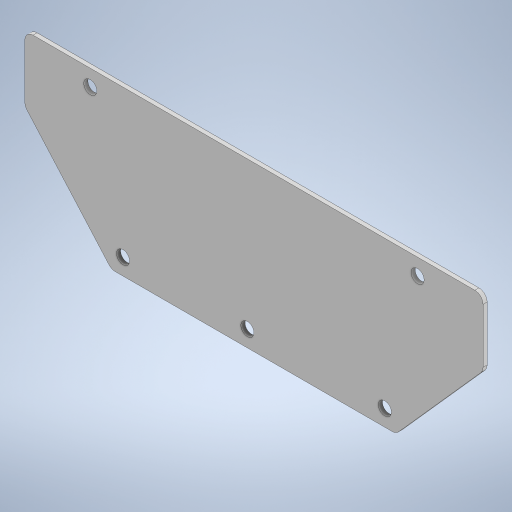
# Autodesk Inventor part: wedge
Saved by Autodesk Inventor 2023.4 (Build 274418000, 418)
## iProperties
Created: 2023-12-11
Part Number: wedge
Material: Generic
Document SubType Name: Modeling
Designer: Meer
Density: 1 g/cm^3
Appearance: Default
Author: Meer
Autodesk Inventor part; units mm, degrees
ref_plane "YZ Plane" through (0, 0, 0) normal (1, 0, 0) x (0, 1, 0)
ref_plane "XZ Plane" through (0, 0, 0) normal (0, 1, 0) x (-1, 0, 0)
ref_plane "XY Plane" through (0, 0, 0) normal (0, 0, 1) x (1, 0, 0)
sketch "Sketch1" plane through (0, 0, 0) normal (0, 0, 1) x (1, 0, 0)
  line L0 (-83.8471, 83.8315) -> (93.9529, 83.8315)
  line L1 (93.9529, 83.8315) -> (93.9529, 20.3315)
  line L2 (93.9529, 20.3315) -> (-83.8471, 20.3315)
  line L3 (-83.8471, 20.3315) -> (-83.8471, 83.8315)
  line L4 (-83.8471, 20.3315) -> (-83.8471, 58.4315)
  line L5 (93.9529, 20.3315) -> (93.9529, 58.2798)
  line L6 (93.9529, 58.2798) -> (60.1807, 20.3315)
  line L7 (-83.8471, 58.4315) -> (-50.246, 20.3315)
  circle A0 centre (-58.4471, 77.4815) radius 2.54
  circle A1 centre (68.5529, 77.4815) radius 2.54
  circle A2 centre (2.5129, 26.6815) radius 2.54
  circle A3 centre (-45.7471, 26.6815) radius 2.54
  circle A4 centre (55.8529, 26.6815) radius 2.54
  point P0 (0, 0)
  dimension "d0" = 177.8
  dimension "d1" = 63.5
  dimension "d2" = 38.1
  dimension "d3" = 50.8
  dimension "d4" = 50.8
  dimension "d18" = 6.35
  dimension "d19" = 25.4
  dimension "d20" = 5.08
  dimension "d21" = 5.08
  dimension "d22" = 6.35
  dimension "d23" = 25.4
  dimension "d24" = 5.08
  dimension "d25" = 6.35
  dimension "d26" = 86.36
  dimension "d29" = 6.35
  dimension "d30" = 6.35
  dimension "d31" = 38.1
  dimension "d32" = 38.1
  dimension "d33" = 5.08
  dimension "d34" = 5.08
  constraints: 16 end point, 5 centre point, 4 point on line, 2 parallel, 1 horizontal, 1 perpendicular
  measures "d0" distance of L0.start L0.end
  measures "d1" distance of L0.end L1.end
  measures "d2" distance of L2.end L4.end
  measures "d3" distance of L5.end L6.end
  measures "d4" distance of L4.end L7.end
  measures "d18" distance from line of L0 A0.centre
  measures "d19" distance from line of L3 A0.centre
  measures "d20" diameter of A0
  measures "d21" diameter of A1
  measures "d22" distance from line of L0 A1.centre
  measures "d23" distance from line of L1 A1.centre
  measures "d24" diameter of A2
  measures "d25" distance from line of L2 A2.centre
  measures "d26" distance from line of L3 A2.centre
  measures "d29" distance from line of L2 A4.centre
  measures "d30" distance from line of L2 A3.centre
  measures "d31" distance from line of L3 A3.centre
  measures "d32" distance from line of L1 A4.centre
  measures "d33" diameter of A3
  measures "d34" diameter of A4
extrude "Extrusion3" add sketch "Sketch1" along normal blind 1.5875 contours L0 L1 L6 L2 L7 L3
fillet "Fillet6" radius 3.175 4 edges at (-83.8471, 58.4315, 0.7937) (-50.246, 20.3315, 0.7937) (60.1807, 20.3315, 0.7937) (-83.8471, 83.8315, 0.7937)
fillet "Fillet7" radius 3.175 2 edges at (93.9529, 83.8315, 0.7937) (93.9529, 58.2798, 0.7937)
body "Solid3"
